frsky_xm_plus (Autodesk Fusion 360 design; units mm, degrees)
Autodesk Fusion 360 part; units mm, degrees
sketch "Sketch1" plane through (0, 0, 0) normal (0, 1, 0) x (1, 0, 0)
  line L0 (6, 10.7875) -> (-6, 10.7875)
  line L1 (-6, 10.7875) -> (-6, -10.7875)
  line L2 (-6, -10.7875) -> (6, -10.7875)
  line L3 (6, -10.7875) -> (6, 10.7875)
  line L4 (6, 10.7875) -> (-6, -10.7875) construction
  line L5 (-6, 10.7875) -> (6, -10.7875) construction
  dimension "d1274" = 21.575
  dimension "d1275" = 12
  dimension "d1788" = 0
  dimension "d1789" = 0
  dimension "d1790" = 0
  dimension "d1791" = 0
  dimension "d2281" = 0
  dimension "d2282" = 0
  dimension "d2283" = 0
  dimension "d2284" = 0
  dimension "d2348" = 0
  dimension "d2349" = 0
  dimension "d2350" = 0
  dimension "d2351" = 0
  dimension "d2418" = 0
  dimension "d2419" = 0
  dimension "d2420" = 0
  dimension "d2421" = 0
  dimension "d2495" = 0
  dimension "d2496" = 0
  dimension "d2497" = 0
  dimension "d2498" = 0
  dimension "d2795" = 0
  dimension "d2796" = 0
  dimension "d2797" = 0
  dimension "d2798" = 0
  measures "d1274" distance of L0.end L1.end
  measures "d1275" distance of L1.end L2.end
extrude "Extrude1" add sketch "Sketch1" along normal blind 4
